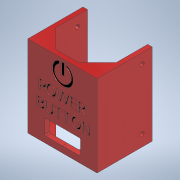
# Autodesk Inventor part: Power Switch Shroud
Saved by Autodesk Inventor 2022 (Build 260153000, 153)
## iProperties
Created: 2022-09-29
Part Number: Power Switch Shroud
Material: Generic
Document SubType Name: Modeling
Designer: matt
Density: 1 g/cm^3
Appearance: Default
Author: matt
Autodesk Inventor part; units mm, degrees
ref_plane "YZ Plane" through (0, 0, 0) normal (1, 0, 0) x (0, 1, 0)
ref_plane "XZ Plane" through (0, 0, 0) normal (0, 1, 0) x (-1, 0, 0)
sketch "Sketch1" plane through (0, 0, 0) normal (0, 0, 1) x (1, 0, 0)
  spline S0 degree 2 poles (16.9746, 22.5367) (16.5733, 22.1785) (15.505, 21.8327) (14.7393, 21.8327) knots 0 0 0 1 2 2 2
  spline S1 degree 2 poles (14.7393, 21.8327) (13.9983, 21.8327) (12.8929, 22.1847) (12.5039, 22.5367) knots 0 0 0 1 2 2 2
  spline S2 degree 2 poles (12.5039, 22.5367) (12.0655, 22.9319) (11.7073, 24.0434) (11.7073, 24.8585) knots 0 0 0 1 2 2 2
  line L0 (11.7073, 24.8585) -> (11.7073, 29.6132)
  line L1 (11.7073, 29.6132) -> (12.8188, 29.6132)
  line L2 (12.8188, 29.6132) -> (12.8188, 24.8585)
  spline S3 degree 2 poles (12.8188, 24.8585) (12.8188, 24.3274) (12.967, 23.6111) (13.177, 23.3209) knots 0 0 0 1 2 2 2
  spline S4 degree 2 poles (13.177, 23.3209) (13.4055, 23.0121) (14.1774, 22.6972) (14.7393, 22.6972) knots 0 0 0 1 2 2 2
  spline S5 degree 2 poles (14.7393, 22.6972) (15.258, 22.6972) (16.0731, 23.0121) (16.3016, 23.3209) knots 0 0 0 1 2 2 2
  spline S6 degree 2 poles (16.3016, 23.3209) (16.5053, 23.6111) (16.6597, 24.3212) (16.6597, 24.8338) knots 0 0 0 1 2 2 2
  line L3 (16.6597, 24.8338) -> (16.6597, 29.6132)
  line L4 (16.6597, 29.6132) -> (17.7712, 29.6132)
  line L5 (17.7712, 29.6132) -> (17.7712, 24.8585)
  spline S7 degree 2 poles (17.7712, 24.8585) (17.7712, 24.0619) (17.4193, 22.9257) (16.9746, 22.5367) knots 0 0 0 1 2 2 2
  line L6 (36.7065, 34.5394) -> (31.4639, 34.5394)
  line L7 (31.4639, 34.5394) -> (31.4639, 42.1594)
  line L8 (31.4639, 42.1594) -> (36.7065, 42.1594)
  line L9 (36.7065, 42.1594) -> (36.7065, 41.2578)
  line L10 (36.7065, 41.2578) -> (32.5754, 41.2578)
  line L11 (32.5754, 41.2578) -> (32.5754, 39.1707)
  line L12 (32.5754, 39.1707) -> (36.4224, 39.1707)
  line L13 (36.4224, 39.1707) -> (36.4224, 38.2691)
  line L14 (36.4224, 38.2691) -> (32.5754, 38.2691)
  line L15 (32.5754, 38.2691) -> (32.5754, 35.4409)
  line L16 (32.5754, 35.4409) -> (36.7065, 35.4409)
  line L17 (36.7065, 35.4409) -> (36.7065, 34.5394)
  line L18 (24.1252, 62.4931) -> (25.3952, 62.4931)
  line L19 (26.6652, 62.4931) -> (26.6652, 53.0031)
  line L20 (26.6652, 53.0031) -> (24.1252, 53.0031)
  line L21 (24.1252, 53.0031) -> (24.1252, 62.4931)
  arc A0 (22.768, 60.1792) -> (27.8481, 60.253) centre (25.3952, 54.2179) ccw
  line L22 (27.8481, 60.253) -> (27.8485, 62.29)
  arc A1 (22.7685, 62.2948) -> (27.8485, 62.29) centre (25.3009, 54.1994) ccw
  line L23 (22.7685, 62.2948) -> (22.768, 60.1792)
  spline S8 degree 2 poles (10.8578, 41.6839) (11.3209, 41.3937) (11.852, 40.4983) (11.852, 39.8623) knots 0 0 0 1 2 2 2
  spline S9 degree 2 poles (11.852, 39.8623) (11.852, 39.3683) (11.4629, 38.4791) (11.1233, 38.1703) knots 0 0 0 1 2 2 2
  spline S10 degree 2 poles (11.1233, 38.1703) (10.6849, 37.7813) (9.5178, 37.3799) (8.6224, 37.3799) knots 0 0 0 1 2 2 2
  line L24 (8.6224, 37.3799) -> (7.6776, 37.3799)
  line L25 (7.6776, 37.3799) -> (7.6776, 34.5394)
  line L26 (7.6776, 34.5394) -> (6.5661, 34.5394)
  line L27 (6.5661, 34.5394) -> (6.5661, 42.1594)
  line L28 (6.5661, 42.1594) -> (8.6718, 42.1594)
  spline S11 degree 2 poles (8.6718, 42.1594) (9.4128, 42.1594) (10.4564, 41.9371) (10.8578, 41.6839) knots 0 0 0 1 2 2 2
  spline S12 degree 2 poles (16.1436, 42.3199) (16.9958, 42.3199) (18.3666, 41.7765) (18.8421, 41.2887) knots 0 0 0 1 2 2 2
  spline S13 degree 2 poles (18.8421, 41.2887) (19.3176, 40.7823) (19.8486, 39.3003) (19.8486, 38.3494) knots 0 0 0 1 2 2 2
  spline S14 degree 2 poles (19.8486, 38.3494) (19.8486, 37.4231) (19.3299, 35.9226) (18.8421, 35.4162) knots 0 0 0 1 2 2 2
  spline S15 degree 2 poles (18.8421, 35.4162) (18.3296, 34.8852) (16.9649, 34.3788) (16.1436, 34.3788) knots 0 0 0 1 2 2 2
  spline S16 degree 2 poles (16.1436, 34.3788) (15.2915, 34.3788) (13.9268, 34.9037) (13.4389, 35.4162) knots 0 0 0 1 2 2 2
  spline S17 degree 2 poles (13.4389, 35.4162) (12.9573, 35.9226) (12.4386, 37.4108) (12.4386, 38.3494) knots 0 0 0 1 2 2 2
  spline S18 degree 2 poles (12.4386, 38.3494) (12.4386, 39.3065) (12.9635, 40.7638) (13.4451, 41.2887) knots 0 0 0 1 2 2 2
  spline S19 degree 2 poles (13.4451, 41.2887) (13.9268, 41.7951) (15.2976, 42.3199) (16.1436, 42.3199) knots 0 0 0 1 2 2 2
  line L29 (29.3767, 42.1594) -> (30.4635, 42.1594)
  line L30 (30.4635, 42.1594) -> (28.3578, 34.5394)
  line L31 (28.3578, 34.5394) -> (27.1105, 34.5394)
  line L32 (27.1105, 34.5394) -> (25.4, 40.8626)
  line L33 (25.4, 40.8626) -> (23.7451, 34.5394)
  line L34 (23.7451, 34.5394) -> (22.5101, 34.5394)
  line L35 (22.5101, 34.5394) -> (20.3673, 42.1594)
  line L36 (20.3673, 42.1594) -> (21.5159, 42.1594)
  line L37 (21.5159, 42.1594) -> (23.2017, 35.8361)
  line L38 (23.2017, 35.8361) -> (24.8751, 42.1594)
  line L39 (24.8751, 42.1594) -> (26.0052, 42.1594)
  line L40 (26.0052, 42.1594) -> (27.6971, 35.7559)
  line L41 (27.6971, 35.7559) -> (29.3767, 42.1594)
  line L42 (41.4304, 37.8554) -> (44.4129, 34.5394)
  line L43 (44.4129, 34.5394) -> (42.968, 34.5394)
  line L44 (42.968, 34.5394) -> (40.3127, 37.5713)
  line L45 (40.3127, 37.5713) -> (39.0407, 37.5713)
  line L46 (39.0407, 37.5713) -> (39.0407, 34.5394)
  line L47 (39.0407, 34.5394) -> (37.9292, 34.5394)
  line L48 (37.9292, 34.5394) -> (37.9292, 42.1594)
  line L49 (37.9292, 42.1594) -> (40.0904, 42.1594)
  spline S20 degree 2 poles (40.0904, 42.1594) (40.8067, 42.1594) (41.7824, 42.0174) (42.2208, 41.758) knots 0 0 0 1 2 2 2
  spline S21 degree 2 poles (42.2208, 41.758) (42.6592, 41.4986) (43.1718, 40.6897) (43.1718, 40.0907) knots 0 0 0 1 2 2 2
  spline S22 degree 2 poles (43.1718, 40.0907) (43.1718, 39.2571) (42.2393, 38.1271) (41.4304, 37.8554) knots 0 0 0 1 2 2 2
  spline S23 degree 2 poles (9.1323, 26.2293) (9.8795, 26.0441) (10.7008, 25.0623) (10.7008, 24.3336) knots 0 0 0 1 2 2 2
  spline S24 degree 2 poles (10.7008, 24.3336) (10.7008, 23.7655) (10.2253, 22.8948) (9.8301, 22.6108) knots 0 0 0 1 2 2 2
  spline S25 degree 2 poles (9.8301, 22.6108) (9.3546, 22.2773) (8.274, 21.9932) (7.4219, 21.9932) knots 0 0 0 1 2 2 2
  line L50 (7.4219, 21.9932) -> (5.0198, 21.9932)
  line L51 (5.0198, 21.9932) -> (5.0198, 29.6132)
  line L52 (5.0198, 29.6132) -> (7.2428, 29.6132)
  spline S26 degree 2 poles (7.2428, 29.6132) (8.1382, 29.6132) (9.0274, 29.5083) (9.4411, 29.3045) knots 0 0 0 1 2 2 2
  spline S27 degree 2 poles (9.4411, 29.3045) (9.8919, 29.0884) (10.3056, 28.3782) (10.3056, 27.8966) knots 0 0 0 1 2 2 2
  spline S28 degree 2 poles (10.3056, 27.8966) (10.3056, 27.3594) (9.6819, 26.5072) (9.1323, 26.2664) knots 0 0 0 1 2 2 2
  line L53 (9.1323, 26.2664) -> (9.1323, 26.2293)
  line L54 (22.4396, 21.9932) -> (21.3281, 21.9932)
  line L55 (21.3281, 21.9932) -> (21.3281, 28.7117)
  line L56 (21.3281, 28.7117) -> (18.5122, 28.7117)
  line L57 (18.5122, 28.7117) -> (18.5122, 29.6132)
  line L58 (18.5122, 29.6132) -> (31.9862, 29.6132)
  line L59 (31.9862, 29.6132) -> (31.9862, 28.7117)
  line L60 (31.9862, 28.7117) -> (29.1704, 28.7117)
  line L61 (29.1704, 28.7117) -> (29.1704, 21.9932)
  line L62 (29.1704, 21.9932) -> (28.0588, 21.9932)
  line L63 (28.0588, 21.9932) -> (28.0588, 28.7117)
  line L64 (28.0588, 28.7117) -> (22.4396, 28.7117)
  line L65 (22.4396, 28.7117) -> (22.4396, 21.9932)
  spline S29 degree 2 poles (36.0555, 29.7738) (36.9077, 29.7738) (38.2785, 29.2304) (38.754, 28.7426) knots 0 0 0 1 2 2 2
  spline S30 degree 2 poles (38.754, 28.7426) (39.2295, 28.2362) (39.7605, 26.7542) (39.7605, 25.8032) knots 0 0 0 1 2 2 2
  spline S31 degree 2 poles (39.7605, 25.8032) (39.7605, 24.877) (39.2418, 23.3765) (38.754, 22.8701) knots 0 0 0 1 2 2 2
  spline S32 degree 2 poles (38.754, 22.8701) (38.2415, 22.339) (36.8768, 21.8327) (36.0555, 21.8327) knots 0 0 0 1 2 2 2
  spline S33 degree 2 poles (36.0555, 21.8327) (35.2034, 21.8327) (33.8387, 22.3576) (33.3509, 22.8701) knots 0 0 0 1 2 2 2
  spline S34 degree 2 poles (33.3509, 22.8701) (32.8692, 23.3765) (32.3505, 24.8646) (32.3505, 25.8032) knots 0 0 0 1 2 2 2
  spline S35 degree 2 poles (32.3505, 25.8032) (32.3505, 26.7604) (32.8754, 28.2177) (33.357, 28.7426) knots 0 0 0 1 2 2 2
  spline S36 degree 2 poles (33.357, 28.7426) (33.8387, 29.2489) (35.2095, 29.7738) (36.0555, 29.7738) knots 0 0 0 1 2 2 2
  line L66 (46.973, 29.6132) -> (46.973, 21.9932)
  line L67 (46.973, 21.9932) -> (45.7195, 21.9932)
  line L68 (45.7195, 21.9932) -> (42.0268, 28.5635)
  line L69 (42.0268, 28.5635) -> (42.0268, 21.9932)
  line L70 (42.0268, 21.9932) -> (40.9832, 21.9932)
  line L71 (40.9832, 21.9932) -> (40.9832, 29.6132)
  line L72 (40.9832, 29.6132) -> (42.564, 29.6132)
  line L73 (42.564, 29.6132) -> (45.9294, 23.5802)
  line L74 (45.9294, 23.5802) -> (45.9294, 29.6132)
  line L75 (45.9294, 29.6132) -> (46.973, 29.6132)
  line L76 (52.8952, 65) -> (-2.1048, 65)
  line L77 (-2.1048, 65) -> (-2.1048, 0)
  line L78 (-2.1048, 0) -> (52.8952, 0)
  line L79 (52.8952, 0) -> (52.8952, 65)
  arc A2 (12.3101, 17.3013) -> (11.3108, 16.3013) centre (12.3108, 16.3013) ccw
  line L80 (12.3101, 17.3013) -> (25.3952, 17.3095)
  arc A3 (39.8108, 16.3024) -> (38.4803, 17.2742) centre (38.8112, 16.3305) ccw
  line L81 (39.8108, 16.3024) -> (39.8108, 6.0206)
  arc A4 (38.4803, 5.0177) -> (39.8108, 6.0206) centre (38.8126, 5.9609) ccw
  line L82 (38.4803, 5.0177) -> (25.3952, 5.0095)
  arc A5 (11.3108, 6) -> (12.3102, 5) centre (12.3108, 6) ccw
  line L83 (11.3108, 6) -> (11.3108, 16.3013)
  spline S37 degree 2 poles (18.0023, 40.6527) (17.6688, 41.0479) (16.7302, 41.4431) (16.1436, 41.4431) knots 0 0 0 1 2 2 2
  spline S38 degree 2 poles (16.1436, 41.4431) (15.5385, 41.4431) (14.6369, 41.0602) (14.2849, 40.6527) knots 0 0 0 1 2 2 2
  spline S39 degree 2 poles (14.2849, 40.6527) (13.9515, 40.2636) (13.5995, 39.0904) (13.5995, 38.3494) knots 0 0 0 1 2 2 2
  spline S40 degree 2 poles (13.5995, 38.3494) (13.5995, 36.8488) (14.9827, 35.2557) (16.1436, 35.2557) knots 0 0 0 1 2 2 2
  spline S41 degree 2 poles (16.1436, 35.2557) (17.3107, 35.2557) (18.6877, 36.8488) (18.6877, 38.3494) knots 0 0 0 1 2 2 2
  spline S42 degree 2 poles (18.6877, 38.3494) (18.6877, 39.1027) (18.3296, 40.2698) (18.0023, 40.6527) knots 0 0 0 1 2 2 2
  spline S43 degree 2 poles (10.0921, 40.9923) (9.8265, 41.1528) (9.1226, 41.2825) (8.5977, 41.2825) knots 0 0 0 1 2 2 2
  line L84 (8.5977, 41.2825) -> (7.6776, 41.2825)
  line L85 (7.6776, 41.2825) -> (7.6776, 38.2444)
  line L86 (7.6776, 38.2444) -> (8.4372, 38.2444)
  spline S44 degree 2 poles (8.4372, 38.2444) (9.1102, 38.2444) (9.9439, 38.442) (10.2218, 38.7014) knots 0 0 0 1 2 2 2
  spline S45 degree 2 poles (10.2218, 38.7014) (10.4688, 38.9298) (10.6911, 39.4671) (10.6911, 39.8314) knots 0 0 0 1 2 2 2
  spline S46 degree 2 poles (10.6911, 39.8314) (10.6911, 40.2266) (10.3946, 40.807) (10.0921, 40.9923) knots 0 0 0 1 2 2 2
  spline S47 degree 2 poles (41.4798, 41.0232) (41.2452, 41.1652) (40.6153, 41.2825) (40.146, 41.2825) knots 0 0 0 1 2 2 2
  line L87 (40.146, 41.2825) -> (39.0407, 41.2825)
  line L88 (39.0407, 41.2825) -> (39.0407, 38.4173)
  line L89 (39.0407, 38.4173) -> (40.0225, 38.4173)
  spline S48 degree 2 poles (40.0225, 38.4173) (40.498, 38.4173) (41.2699, 38.5717) (41.5354, 38.8125) knots 0 0 0 1 2 2 2
  spline S49 degree 2 poles (41.5354, 38.8125) (41.7824, 39.0225) (42.0109, 39.6153) (42.0109, 40.0105) knots 0 0 0 1 2 2 2
  spline S50 degree 2 poles (42.0109, 40.0105) (42.0109, 40.3439) (41.7515, 40.8564) (41.4798, 41.0232) knots 0 0 0 1 2 2 2
  spline S51 degree 2 poles (37.9142, 28.1065) (37.5808, 28.5017) (36.6422, 28.8969) (36.0555, 28.8969) knots 0 0 0 1 2 2 2
  spline S52 degree 2 poles (36.0555, 28.8969) (35.4504, 28.8969) (34.5488, 28.5141) (34.1968, 28.1065) knots 0 0 0 1 2 2 2
  spline S53 degree 2 poles (34.1968, 28.1065) (33.8634, 27.7175) (33.5114, 26.5443) (33.5114, 25.8032) knots 0 0 0 1 2 2 2
  spline S54 degree 2 poles (33.5114, 25.8032) (33.5114, 24.3027) (34.8946, 22.7096) (36.0555, 22.7096) knots 0 0 0 1 2 2 2
  spline S55 degree 2 poles (36.0555, 22.7096) (37.2226, 22.7096) (38.5996, 24.3027) (38.5996, 25.8032) knots 0 0 0 1 2 2 2
  spline S56 degree 2 poles (38.5996, 25.8032) (38.5996, 26.5566) (38.2415, 27.7237) (37.9142, 28.1065) knots 0 0 0 1 2 2 2
  spline S57 degree 2 poles (8.7186, 28.5511) (8.4469, 28.687) (7.7862, 28.7487) (7.1996, 28.7487) knots 0 0 0 1 2 2 2
  line L90 (7.1996, 28.7487) -> (6.1313, 28.7487)
  line L91 (6.1313, 28.7487) -> (6.1313, 26.5196)
  line L92 (6.1313, 26.5196) -> (7.3972, 26.5196)
  spline S58 degree 2 poles (7.3972, 26.5196) (7.922, 26.5196) (8.416, 26.6184) (8.6754, 26.7727) knots 0 0 0 1 2 2 2
  spline S59 degree 2 poles (8.6754, 26.7727) (8.9286, 26.9209) (9.1447, 27.3964) (9.1447, 27.7546) knots 0 0 0 1 2 2 2
  spline S60 degree 2 poles (9.1447, 27.7546) (9.1447, 28.0263) (8.9409, 28.4338) (8.7186, 28.5511) knots 0 0 0 1 2 2 2
  spline S61 degree 2 poles (8.8606, 25.476) (8.5951, 25.5995) (7.9714, 25.6736) (7.3972, 25.6736) knots 0 0 0 1 2 2 2
  line L93 (7.3972, 25.6736) -> (6.1313, 25.6736)
  line L94 (6.1313, 25.6736) -> (6.1313, 22.8578)
  line L95 (6.1313, 22.8578) -> (7.039, 22.8578)
  spline S62 degree 2 poles (7.039, 22.8578) (7.7677, 22.8578) (8.6136, 22.9813) (8.9347, 23.1789) knots 0 0 0 1 2 2 2
  spline S63 degree 2 poles (8.9347, 23.1789) (9.2497, 23.3826) (9.5399, 23.889) (9.5399, 24.2904) knots 0 0 0 1 2 2 2
  spline S64 degree 2 poles (9.5399, 24.2904) (9.5399, 24.7226) (9.2682, 25.2784) (8.8606, 25.476) knots 0 0 0 1 2 2 2
  line L96 (25.3952, 65) -> (25.3952, 0) construction
  line L97 (25.3952, 62.4931) -> (26.6652, 62.4931)
  line L98 (25.3952, 17.3095) -> (38.4803, 17.2742)
  line L99 (25.3952, 5.0095) -> (12.3102, 5)
  line L100 (-2.1048, 0) -> (1.3952, 0)
  line L101 (1.3952, 0) -> (1.3952, 65)
  line L102 (1.3952, 65) -> (-2.1048, 65)
  line L103 (-2.1048, 65) -> (-2.1048, 0)
  line L104 (52.8952, 0) -> (49.3952, 0)
  line L105 (49.3952, 0) -> (49.3952, 65)
  line L106 (49.3952, 65) -> (52.8952, 65)
  line L107 (52.8952, 65) -> (52.8952, 0)
  point P0 (0, 0)
  point P1 (49.3952, 0)
  point P2 (1.3952, 0)
  dimension "d0" = 2.54
  dimension "d1" = 9.49
  dimension "d2" = 5.08
  dimension "d3" = 1.8716
  dimension "d4" = 6.5145
  dimension "d6" = 12.3
  dimension "d8" = 65
  dimension "d11" = 1
  dimension "d12" = 28.5
  dimension "d13" = 3.5
  dimension "d14" = 3.5
  dimension "d44" = 48
  constraints: 216 end point, 12 point on circle, 7 parallel, 6 centre point, 6 point on line, 5 perpendicular, 4 equal length, 3 equal radius, 2 horizontal, 2 midpoint, 2 tangent, 195 other
  measures "d0" distance between parallel lines of L19 L21
  measures "d1" distance between parallel lines of L20 L18
  measures "d2" distance between parallel lines of L22 L23
  measures "d4" radius of A0
  measures "d6" distance between parallel lines of L82 L80
  measures "d8" distance between parallel lines of L78 L76
  measures "d11" radius of A3
  measures "d12" distance between parallel lines of L81 L83
  measures "d13" distance of L102.end L101.end
  measures "d14" distance of L105.end L106.end
  measures "d44" distance between parallel lines of L105 L101
extrude "Extrusion1" add sketch "Sketch1" along normal blind 3 contours S0 S1 S2 L0 L1 L2 S3 S4 S5 S6 L3 L4 L5 S7 | L6 L7 L8 L9 L10 L11 L12 L13 L14 L15 L16 L17 | L18 L97 L19 L20 L21 | A0 L22 A1 L23 | S8 S9 S10 L24 L25 L26 L27 L28 S11 | S12 S13 S14 S15 S16 S17 S18 S19 | L29 L30 L31 L32 L33 L34 L35 L36 L37 L38 L39 L40 L41 | L42 L43 L44 L45 L46 L47 L48 L49 S20 S21 S22 | S23 S24 S25 L50 L51 L52 S26 S27 S28 L53 | L54 L55 L56 L57 L58 L59 L60 L61 L62 L63 L64 L65 | S29 S30 S31 S32 S33 S34 S35 S36 | L66 L67 L68 L69 L70 L71 L72 L73 L74 L75 | L79 L78 L105 L76 | L105 L78 L101 L76 | L101 L78 L77 L76 | S42 S41 S40 S39 S38 S37 | S46 S45 S44 L86 L85 L84 S43 | S50 S49 S48 L89 L88 L87 S47 | S56 S55 S54 S53 S52 S51 | S60 S59 S58 L92 L91 L90 S57 | S64 S63 S62 L95 L94 L93 S61
extrude "Extrusion2" add sketch "Sketch1" along normal blind 0.8 from surface at 3
extrude "Extrusion3" add sketch "Sketch1" against normal blind 40 contours L79 L78 L105 L76 | L101 L78 L77 L76
sketch "Sketch2" plane through (52.8952, 0, 3.8) normal (1, 0, 0) x (0, 0, -1)
  circle A0 centre (35.8, 57) radius 1.8
  line L0 (0, 65) -> (0, 0) projected
  line L1 (43.8, 0) -> (0, 0) projected
  line L2 (43.8, 65) -> (43.8, 0) projected
  line L3 (0, 65) -> (43.8, 65) projected
  circle A1 centre (35.8, 9) radius 1.8
  point P0 (3.8, 0)
  dimension "d21" = 8
  dimension "d22" = 8
  dimension "d25" = 48
  dimension "d32" = 3.6
  constraints: 2 centre point, 1 vertical, 2 other
  measures "d21" distance from line of L2 A0.centre
  measures "d22" distance from line of L3 A0.centre
  measures "d25" distance of A0.centre A1.centre
  measures "d32" diameter of A0
extrude "Extrusion4" cut sketch "Sketch2" against normal through all contours A0 | A1
sketch "Sketch3" plane through (-2.1048, 65, 3.8) normal (0, 1, 0) x (1, 0, 0)
  line L0 (0, 0) -> (55, 0) projected
  line L1 (55, 0) -> (55, 43.8) projected
  line L2 (51.5, 43.8) -> (55, 43.8) projected
  line L3 (51.5, 3.8) -> (51.5, 43.8) projected
  line L4 (51.5, 3.8) -> (3.5, 3.8) projected
  line L5 (3.5, 3.8) -> (3.5, 43.8) projected
  line L6 (0, 43.8) -> (3.5, 43.8) projected
  line L7 (0, 43.8) -> (0, 0) projected
  line L8 (3.5, 3.8) -> (3.5, 43.8) projected
  line L9 (27.5, 4.9802) -> (27.5, 38.1) construction
  line L10 (3.5, 3.8) -> (18.5, 3.8) construction
  line L11 (18.5, 3.8) -> (18.5, 18.8) construction
  line L12 (18.5, 18.8) -> (3.5, 18.8) construction
  line L13 (3.5, 18.8) -> (3.5, 3.8) construction
  line L14 (3.5, 18.8) -> (18.5, 3.8)
  line L15 (51.5, 18.8) -> (36.5, 3.8)
  point P0 (2.1048, 3.8)
  point P1 (14.4149, 3.8)
  point P2 (51.5, 18.8)
  point P3 (36.5, 3.8)
  point P4 (18.5, 3.8)
  point P5 (3.5, 18.8)
  dimension "d33" = 55
  dimension "d34" = 27.5
  dimension "d35" = 15
  dimension "d36" = 15
  constraints: 14 end point, 2 parallel, 2 perpendicular, 2 symmetric about line, 1 horizontal
  measures "d33" distance of L0.start L0.end
  measures "d34" distance between parallel lines of L9 L7
  measures "d35" distance of L12.end L11.end
  measures "d36" distance of L11.end L10.end
extrude "Extrusion5" add sketch "Sketch3" against normal blind 10 contours L14 L4 L5 | L3 L4 L15
extrude "Extrusion6" add sketch "Sketch3" along normal blind 5 from surface at -65 contours L14 L4 L5 | L3 L4 L15
ref_plane "Work Plane1" through (-2.1048, 40, 3.8) normal (0, 1, 0) x (1, 0, 0)
extrude "Extrusion7" add sketch "Sketch3" against normal blind 10 from surface at -25 contours L14 L4 L5 | L3 L4 L15
equation "\"d14\" = d13"
body "Solid1"
